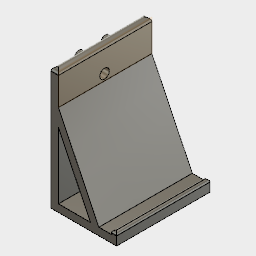
v01 v9 (Autodesk Fusion 360 design; units mm, degrees)
Autodesk Fusion 360 part; units mm, degrees
note: some values were not read from the file. Chosen so that the rebuilt part matches the saved one: which face or edge a step refers to; that a step has no effect.
box "BoxPrimitive1" add length 74 width 49 height 97 placed x (0, 0, -1) y (-1, 0, 0) z (0, 1, 0) at (49, 0, 0) makes body 1
sketch "Sketch2" plane through (0, 0, 0) normal (0, 0, 1) x (1, 0, 0)
  line L0 (0, 97) -> (0, 0)
  line L1 (0, 0) -> (49, 0)
  line L2 (49, 0) -> (49, 97)
  line L3 (49, 97) -> (0, 97)
  line L4 (0, 0) -> (0, 72)
  line L5 (0, 72) -> (6, 72)
  line L6 (0, 0) -> (49, 0)
  line L7 (49, 0) -> (49, 9)
  line L8 (49, 9) -> (45, 9)
  line L9 (45, 9) -> (45, 6)
  line L10 (45, 6) -> (38, 6)
  line L11 (6, 72) -> (38, 6)
  line L12 (0, 72) -> (0, 97)
  line L13 (0, 97) -> (6, 97)
  line L14 (6, 97) -> (6, 72)
  line L15 (45, 9) -> (48, 9)
  line L16 (48, 9) -> (48, 6)
  line L17 (48, 6) -> (45, 6)
  line L18 (45, 6) -> (45, 9)
  dimension "d6" = 72
  dimension "d7" = 6
  dimension "d8" = 9
  dimension "d9" = 4
  dimension "d10" = 3
  dimension "d11" = 7
  dimension "d12" = 25
  dimension "d13" = 6
  measures "d6" distance of L0.end L4.end
  measures "d7" distance of L4.end L5.end
  measures "d8" distance of L1.end L7.end
  measures "d9" distance of L7.end L8.end
  measures "d10" distance of L8.end L9.end
  measures "d11" distance of L9.end L10.end
  measures "d12" distance of L4.end L0.start
  measures "d13" distance of L0.start L13.end
extrude "Extrude4" cut sketch "Sketch2" against normal blind 90 contours L8 L9 L15 L16 L17 L18 bodies 1
extrude "Extrude1" cut sketch "Sketch2" against normal blind 75 contours L2 L3 L8 L9 L10 L11 L14 L15 L18 bodies 1
shell "Shell1" thickness 6 removed faces 1 at (14.6667, 26, 0) on bodies 1
sketch "Sketch3" plane through (0, 0, 0) normal (0, 0, 1) x (1, 0, 0)
  line L0 (6, 6) -> (6, 58.2472)
  line L1 (6, 6) -> (31.332, 6)
  line L2 (31.332, 6) -> (6, 58.2472)
  line L3 (31.332, 6) -> (6, 6)
  point P0 (6, 6)
  point P1 (31.332, 6)
extrude "Extrude2" cut sketch "Sketch3" against normal blind 110 bodies 1
sketch "Sketch4" plane through (6, 0, 0) normal (1, 0, 0) x (0, 0, -1)
  line L0 (74, 72) -> (74, 97)
  line L1 (74, 97) -> (0, 97)
  line L2 (0, 97) -> (0, 72)
  line L3 (0, 72) -> (74, 72)
sketch "Sketch5" plane through (49, 0, 0) normal (1, 0, 0) x (0, 0, -1)
  line L0 (74, 9) -> (0, 9)
  line L1 (0, 9) -> (0, 0)
  line L2 (0, 0) -> (74, 0)
  line L3 (74, 0) -> (74, 9)
  line L4 (0, 9) -> (74, 9)
  line L5 (74, 9) -> (74, 0)
  line L6 (74, 0) -> (0, 0)
  line L7 (0, 0) -> (0, 9)
extrude "Extrude3" add sketch "Sketch5" along normal blind 3 bodies 1
sketch "Sketch6" plane through (0, 0, 0) normal (-1, 0, 0) x (0, 0, 1)
  line L0 (-74, 97) -> (-74, 0)
  line L1 (-74, 0) -> (0, 0)
  line L2 (0, 0) -> (0, 97)
  line L3 (0, 97) -> (-74, 97)
  line L4 (-74, 97) -> (-47, 97)
  line L5 (-47, 97) -> (-47, 90)
  line L6 (-47, 90) -> (-74, 90)
  line L7 (-74, 90) -> (-74, 97)
  line L8 (-47, 90) -> (-26, 90)
  line L9 (-26, 90) -> (-26, 77)
  line L10 (-26, 77) -> (-47, 77)
  line L11 (-47, 77) -> (-47, 90)
  circle A0 centre (-36.5, 77) radius 3.75
  dimension "d23" = 27
  dimension "d24" = 21
  dimension "d25" = 13
  dimension "d46" = 7.5
  measures "d23" distance of L0.start L4.end
  measures "d24" distance of L5.end L8.end
  measures "d25" distance of L5.end L10.end
  measures "d46" diameter of A0
extrude "Extrude9" cut sketch "Sketch6" against normal blind 12 contours L10 A0 | L10 A0 bodies 1
cylinder "CylinderPrimitive1" add diameter 7 height 3.9 placed x (0, 0, 1) y (0, 1, 0) z (-1, 0, 0) at (0, 90, -47) bodies 1
sketch "Sketch7" plane through (-3.9, 0, 0) normal (-1, 0, 0) x (0, 0, 1)
  circle A0 centre (-47, 90) radius 3.5
  circle A1 centre (-47, 90.2172) radius 1
  line L0 (-47, 97) -> (-47, 90)
  dimension "d28" = 2
  measures "d28" diameter of A1
extrude "Extrude5" cut sketch "Sketch7" against normal blind 3.9 contours A1 bodies 1
cylinder "CylinderPrimitive2" add diameter 7 height 3.9 placed x (0, 0, 1) y (0, 1, 0) z (-1, 0, 0) at (0, 90, -26) bodies 1
sketch "Sketch9" plane through (-3.9, 0, 0) normal (-1, 0, 0) x (0, 0, 1)
  circle A0 centre (-26, 90) radius 3.5
  circle A1 centre (-26, 90) radius 1
  dimension "d33" = 2
  measures "d33" diameter of A1
extrude "Extrude6" cut sketch "Sketch9" against normal blind 3.9 contours A1 bodies 1
cylinder "CylinderPrimitive3" add diameter 7 height 3.9 placed x (0, 0, 1) y (0, 1, 0) z (-1, 0, 0) at (-3.9, 77, -47) separate body makes body 2
cylinder "CylinderPrimitive4" add diameter 7 height 3.9 placed x (0, 0, 1) y (0, 1, 0) z (-1, 0, 0) at (0, 77, -26) bodies 1
sketch "Sketch12" plane through (-7.8, 0, 0) normal (-1, 0, 0) x (0, 0, 1)
  circle A0 centre (-47, 77) radius 3.5
  circle A1 centre (-47, 77) radius 1
  dimension "d40" = 2
  measures "d40" diameter of A1
extrude "Extrude7" cut sketch "Sketch12" against normal blind 3.9 contours A1 bodies 2
move_body "Move1" bodies 2 to x (1, 0, 0) y (0, 1, 0) z (0, 0, 1) at (3.9, 0, 0)
sketch "Sketch13" plane through (-3.9, 0, 0) normal (-1, 0, 0) x (0, 0, 1)
  circle A0 centre (-26, 77) radius 3.5
  circle A1 centre (-26, 77) radius 1
  dimension "d43" = 2
  measures "d43" diameter of A1
extrude "Extrude8" cut sketch "Sketch13" against normal blind 3.9 contours A1 bodies 1
form "Form1" [no effect]
fillet "Fillet1" radius 2 4 edges at (52, 9, -37) (50, 9, -74) (48, 9, -37) (50, 9, 0) on bodies 1
fillet "Fillet2" radius 3 4 edges at (3, 97, -74) (0, 97, -37) (3, 97, 0) (6, 97, -37) on bodies 1
named bodies: "Soporte tornillo"
